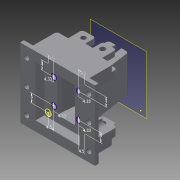
# Autodesk Inventor part: kraken_mount2
Saved by Autodesk Inventor 2014 (Build 180170000, 170)
## iProperties
Created: 2014-01-02
Part Number: kraken_mount2
Material: Generic
Document SubType Name: Modeling
Designer: stephen
Density: 1 g/cm^3
Appearance: Default
Author: stephen
Autodesk Inventor part; units mm, degrees
ref_plane "YZ Plane" through (0, 0, 0) normal (1, 0, 0) x (0, 1, 0)
ref_plane "XZ Plane" through (0, 0, 0) normal (0, 1, 0) x (-1, 0, 0)
ref_plane "XY Plane" through (0, 0, 0) normal (0, 0, 1) x (1, 0, 0)
sketch "Sketch1" plane through (0, 0, 0) normal (0, 1, 0) x (-1, 0, 0)
  line L0 (0, 0) -> (35.3, 0)
  line L1 (35.3, 0) -> (35.3, 40.3)
  line L2 (35.3, 40.3) -> (0, 40.3)
  line L3 (0, 40.3) -> (0, 0)
  line L4 (40.3, 45.3) -> (40.3, -5)
  line L5 (40.3, -5) -> (-5, -5)
  line L6 (-5, -5) -> (-5, 45.3)
  line L7 (-5, 45.3) -> (40.3, 45.3)
  dimension "d0" = 35.3
  dimension "d1" = 40.3
  dimension "d2" = 5
  constraints: 16 end point, 4 parallel, 2 perpendicular, 1 horizontal, 3 other
  measures "d0" distance of L2.end L1.end
  measures "d1" distance of L1.end L0.end
  measures "d2" distance between parallel lines of L6 L3
extrude "Extrusion1" add sketch "Sketch1" along normal blind 8
sketch "Sketch2" plane through (0, 8, 0) normal (0, 1, 0) x (1, 0, 0)
  line L0 (0, 0) -> (0, -40.3) projected
  line L1 (0, -40.3) -> (-35.3, -40.3) projected
  line L2 (-35.3, -40.3) -> (-35.3, 0) projected
  line L3 (-35.3, 0) -> (0, 0) projected
  line L4 (-32.2, -5.9) -> (-32.2, -35.2)
  line L5 (-29.8, -37.6) -> (-5.5, -37.6)
  line L6 (-3.1, -35.2) -> (-3.1, -5.9)
  circle A0 centre (-32.2, -3.5) radius 2.4
  circle A1 centre (-3.1, -3.5) radius 2.4
  circle A2 centre (-3.1, -37.6) radius 2.4
  circle A3 centre (-32.2, -37.6) radius 2.4
  line L7 (-5.5659, -5.5659) -> (-5.5659, -34.7341)
  line L8 (-5.5659, -34.7341) -> (-29.7341, -34.7341)
  line L9 (-29.7341, -34.7341) -> (-29.7341, -5.5659)
  line L10 (-29.7341, -5.5659) -> (-5.5659, -5.5659)
  line L11 (-5.5, -3.5) -> (-5.5659, -3.5)
  line L12 (-29.7341, -3.5) -> (-29.8, -3.5)
  dimension "d6" = 4.8
  dimension "d7" = 4.8
  dimension "d8" = 4.8
  dimension "d9" = 4.8
  dimension "d17" = 5.5659
  constraints: 18 end point, 8 point on circle, 4 centre point, 2 point on line, 3 other
  measures "d6" diameter of A0
  measures "d7" diameter of A1
  measures "d8" diameter of A2
  measures "d9" diameter of A3
  measures "d17" distance between parallel lines of L2 L9
extrude "Extrusion2" add sketch "Sketch2" against normal blind 4
sketch "Sketch3" plane through (0, 0, 0) normal (0, -1, 0) x (1, 0, 0)
  line L0 (-40.3, 45.3) -> (-40.3, -5) projected
  line L1 (-40.3, -5) -> (5, -5) projected
  line L2 (4.73, -7.79) -> (-40.03, -7.79)
  line L3 (-40.03, 48.09) -> (4.73, 48.09)
  line L4 (83.85, 15.65) -> (86.85, 15.65)
  circle A0 centre (25.35, 55.15) radius 2.5
  arc A1 (-22.4416, -21.2786) -> (-24.3582, -19.85) centre (-24.3582, -21.85) ccw
  line L5 (66.85, 24.65) -> (63.85, 24.65)
  line L6 (86.85, 10.65) -> (83.85, 10.65)
  circle A2 centre (25.35, 41.15) radius 2.5
  arc A3 (32.35, 38.15) -> (37.35, 33.15) centre (37.35, 38.15) ccw
  line L7 (2.35, 5.15) -> (2.35, 35.15)
  arc A4 (50.35, 7.15) -> (50.5801, 7.1553) centre (50.35, 12.15) ccw
  line L8 (-37.65, 35.15) -> (-37.65, 5.15)
  arc A5 (48.35, 26.15) -> (48.35, 30.15) centre (48.35, 28.15) ccw
  arc A6 (-22.4416, -21.2786) -> (-12.8584, -21.2786) centre (-17.65, -19.85) ccw
  line L9 (83.85, 43.65) -> (86.85, 43.65)
  line L10 (77.85, 41.65) -> (77.85, 38.15)
  arc A7 (86.85, 38.65) -> (86.85, 43.65) centre (86.85, 41.15) ccw
  line L11 (72.85, 33.15) -> (50.5801, 33.15)
  arc A8 (66.85, 24.65) -> (66.85, 29.65) centre (66.85, 27.15) ccw
  circle A9 centre (-42.65, 40.15) radius 2.1
  circle A10 centre (25.35, -14.85) radius 2.5
  arc A11 (83.85, 15.65) -> (83.85, 10.65) centre (83.85, 13.15) ccw
  line L12 (50.5801, 7.15) -> (72.85, 7.15)
  arc A12 (87.85, -6.35) -> (92.85, -1.35) centre (87.85, -1.35) ccw
  circle A13 centre (7.35, 40.15) radius 2.1
  line L13 (-47.65, 0.15) -> (-47.65, 40.15)
  arc A14 (92.85, 41.65) -> (87.85, 46.65) centre (87.85, 41.65) ccw
  arc A15 (66.85, 10.65) -> (66.85, 15.65) centre (66.85, 13.15) ccw
  line L14 (83.85, 29.65) -> (86.85, 29.65)
  line L15 (66.85, 10.65) -> (63.85, 10.65)
  arc A16 (-12.8584, 61.5786) -> (-10.9418, 60.15) centre (-10.9418, 62.15) ccw
  line L16 (83.85, 1.65) -> (86.85, 1.65)
  arc A17 (63.85, 15.65) -> (63.85, 10.65) centre (63.85, 13.15) ccw
  line L17 (48.35, 14.15) -> (38.35, 14.15)
  line L18 (-10.9418, 60.15) -> (27.35, 60.15)
  circle A18 centre (7.35, 0.15) radius 2.1
  line L19 (86.85, -3.35) -> (83.85, -3.35)
  line L20 (92.85, -1.35) -> (92.85, 41.65)
  arc A19 (86.85, -3.35) -> (86.85, 1.65) centre (86.85, -0.85) ccw
  line L21 (38.35, 10.15) -> (48.35, 10.15)
  arc A20 (82.85, 46.65) -> (77.85, 41.65) centre (82.85, 41.65) ccw
  arc A21 (86.85, 24.65) -> (86.85, 29.65) centre (86.85, 27.15) ccw
  line L22 (27.35, -19.85) -> (-10.9418, -19.85)
  arc A22 (-27.65, 60.15) -> (-47.65, 40.15) centre (-27.65, 40.15) ccw
  arc A23 (-10.9418, -19.85) -> (-12.8584, -21.2786) centre (-10.9418, -21.85) ccw
  line L23 (87.85, 46.65) -> (82.85, 46.65)
  arc A24 (48.35, 10.15) -> (48.35, 14.15) centre (48.35, 12.15) ccw
  circle A25 centre (-17.65, -19.85) radius 2.6
  line L24 (32.35, -14.85) -> (32.35, 2.15)
  arc A26 (83.85, 1.65) -> (83.85, -3.35) centre (83.85, -0.85) ccw
  arc A27 (86.85, 10.65) -> (86.85, 15.65) centre (86.85, 13.15) ccw
  circle A28 centre (25.35, 27.15) radius 2.5
  arc A29 (37.35, 7.15) -> (32.35, 2.15) centre (37.35, 2.15) ccw
  circle A30 centre (25.35, -0.85) radius 2.5
  line L25 (-27.65, 60.15) -> (-24.3582, 60.15)
  line L26 (-24.3582, -19.85) -> (-27.65, -19.85)
  line L27 (38.35, 26.15) -> (48.35, 26.15)
  circle A31 centre (-37.65, -12.85) radius 1.75
  line L28 (50.5801, 33.15) -> (50.5801, 33.1447)
  arc A32 (-17.8261, 55.1531) -> (-18.8441, 55.2947) centre (-17.65, 60.15) ccw
  arc A33 (72.85, 33.15) -> (77.85, 38.15) centre (72.85, 38.15) ccw
  arc A34 (38.35, 14.15) -> (38.35, 10.15) centre (38.35, 12.15) ccw
  arc A35 (83.85, 43.65) -> (83.85, 38.65) centre (83.85, 41.15) ccw
  line L29 (82.85, -6.35) -> (87.85, -6.35)
  circle A36 centre (2.35, 53.15) radius 1.75
  arc A37 (2.35, 35.15) -> (-37.65, 35.15) centre (-17.65, 35.15) ccw
  arc A38 (50.5801, 33.1447) -> (50.35, 33.15) centre (50.35, 28.15) ccw
  arc A39 (63.85, 29.65) -> (63.85, 24.65) centre (63.85, 27.15) ccw
  circle A40 centre (25.35, 13.15) radius 2.5
  arc A41 (77.85, -1.35) -> (82.85, -6.35) centre (82.85, -1.35) ccw
  circle A42 centre (-42.65, 20.15) radius 2.1
  arc A43 (-24.3582, 60.15) -> (-22.4416, 61.5786) centre (-24.3582, 62.15) ccw
  arc A44 (38.35, 30.15) -> (38.35, 26.15) centre (38.35, 28.15) ccw
  arc A45 (83.85, 29.65) -> (83.85, 24.65) centre (83.85, 27.15) ccw
  line L30 (50.35, 33.15) -> (37.35, 33.15)
  line L31 (50.35, 7.15) -> (37.35, 7.15)
  arc A46 (27.35, -19.85) -> (32.35, -14.85) centre (27.35, -14.85) ccw
  line L32 (86.85, 24.65) -> (83.85, 24.65)
  line L33 (50.5801, 7.1553) -> (50.5801, 7.15)
  circle A47 centre (7.35, 20.15) radius 2.1
  arc A48 (-37.65, 5.15) -> (2.35, 5.15) centre (-17.65, 5.15) ccw
  line L34 (63.85, 29.65) -> (66.85, 29.65)
  line L35 (48.35, 30.15) -> (38.35, 30.15)
  line L36 (77.85, 2.15) -> (77.85, -1.35)
  circle A49 centre (-17.65, 60.15) radius 2.6
  circle A50 centre (48.35, 20.15) radius 1.25
  line L37 (63.85, 15.65) -> (66.85, 15.65)
  arc A51 (-47.65, 0.15) -> (-27.65, -19.85) centre (-27.65, 0.15) ccw
  circle A52 centre (2.35, -12.85) radius 1.75
  arc A53 (32.35, 55.15) -> (27.35, 60.15) centre (27.35, 55.15) ccw
  arc A54 (77.85, 2.15) -> (72.85, 7.15) centre (72.85, 2.15) ccw
  circle A55 centre (-37.65, 53.15) radius 1.75
  circle A56 centre (-42.65, 0.15) radius 2.1
  line L38 (32.35, 38.15) -> (32.35, 55.15)
  line L39 (86.85, 38.65) -> (83.85, 38.65)
  circle A57 centre (38.35, 20.15) radius 1.25
  line L40 (-40.03, 48.09) -> (-47.6486, 48.09)
  line L41 (-47.6486, 48.09) -> (-47.6486, -7.79)
  line L42 (-47.6486, -7.79) -> (-40.03, -7.79)
  line L43 (4.73, 48.09) -> (12.35, 48.09)
  line L44 (12.35, 48.09) -> (12.35, -7.79)
  line L45 (12.35, -7.79) -> (4.73, -7.79)
  circle A58 centre (7.35, 40.15) radius 2.1
  circle A59 centre (7.35, 20.15) radius 2.1
  circle A60 centre (7.35, 0.15) radius 2.1
  circle A61 centre (-42.65, 40.15) radius 2.1
  circle A62 centre (-42.65, 0.15) radius 2.1
  circle A63 centre (-42.65, 20.15) radius 2.1
  line L46 (-40.3, 45.3) -> (5, 45.3)
  line L47 (5, 45.3) -> (5, -5)
  line L48 (5, -5) -> (-40.3, -5)
  line L49 (-40.3, -5) -> (-40.3, 45.3)
  line L50 (-47.6486, 48.09) -> (12.35, 48.09)
  line L51 (12.35, 48.09) -> (12.35, -7.79)
  line L52 (12.35, -7.79) -> (-47.6486, -7.79)
  line L53 (-47.6486, -7.79) -> (-47.6486, 48.09)
  point P0 (6.3945, 46.914)
  dimension "d12" = 7.62
  constraints: 104 end point, 81 tangent, 76 point on circle, 64 centre point, 55 equal radius, 26 parallel, 11 perpendicular, 6 coincident, 4 horizontal, 1 collinear, 1 concentric
  measures "d12" distance of L45.start L45.end
extrude "Extrusion3" add sketch "Sketch3" along normal blind 3 contours L0 L1 A48 L2 L42 A51 L13 A22 L40 L3 A37 L46 | A37 L3 L46 | L1 A48 L2 | A37 L3 L43 L44 L45 L2 A48 L1 L47 L46 | A22 L41 L40 | L42 L41 A51
sketch "Sketch5" plane through (0, -3, 0) normal (0, -1, 0) x (1, 0, 0)
  line L0 (-40.3, 45.3) -> (5, 45.3) projected
  line L1 (5, 45.3) -> (5, -5) projected
  line L2 (5, -5) -> (-40.3, -5) projected
  line L3 (-40.3, -5) -> (-40.3, 45.3) projected
  line L4 (0, 0) -> (-35.3, 0)
  line L5 (-35.3, 0) -> (-35.3, 40.3)
  line L6 (-35.3, 40.3) -> (0, 40.3)
  line L7 (0, 40.3) -> (0, 0)
  dimension "d15" = 35.3
  dimension "d16" = 40.3
  constraints: 8 end point, 2 parallel, 1 horizontal, 1 perpendicular
  measures "d15" distance of L5.end L6.end
  measures "d16" distance of L4.end L5.end
extrude "Extrusion4" add sketch "Sketch5" against normal up to next
sketch "Sketch6" plane through (0, 0, 0) normal (0, 1, 0) x (1, 0, 0)
  line L0 (-40.3, 5) -> (5, 5) projected
  line L1 (-47.6486, 7.79) -> (12.35, 7.79) projected
  line L2 (5, 5) -> (5, 23.7794)
  line L3 (5, 5) -> (23.7794, 5) construction
  line L4 (-40.3, 5) -> (-40.3, 33.7756)
  line L5 (-40.3, 7.79) -> (5, 7.79)
  line L6 (-40.3, 5) -> (5, 5)
  point P0 (0, 0)
  dimension "d20" = 90
  constraints: 10 end point, 4 point on line, 2 perpendicular, 1 collinear, 1 horizontal
  measures "d20" angle of L3 L2
extrude "Extrusion5" add sketch "Sketch6" along normal up to surface (8 mm away)
sketch "Sketch7" plane through (0, 0, 0) normal (0, 1, 0) x (1, 0, 0)
  line L0 (5, -45.3) -> (-40.3, -45.3) projected
  line L1 (12.35, -48.09) -> (-47.6486, -48.09) projected
  line L2 (5, 7.79) -> (12.35, 7.79) projected
  line L3 (-40.3, -45.3) -> (-40.3, -52.0309)
  line L4 (5, -45.3) -> (5, -53.1235)
  line L5 (5, -48.09) -> (-40.3, -48.09)
  line L6 (-40.3, -45.3) -> (5, -45.3)
  point P0 (0, 0)
  constraints: 8 end point, 4 point on line, 1 collinear, 1 parallel, 1 perpendicular
extrude "Extrusion6" add sketch "Sketch7" along normal up to surface (8 mm away)
sketch "Sketch8" plane through (0, 8, 0) normal (0, 1, 0) x (1, 0, 0)
  line L0 (-40.3, 7.79) -> (-40.3, -48.09) projected
  line L1 (5, -48.09) -> (5, 7.79) projected
  line L2 (5, 7.79) -> (-40.3, 7.79) projected
  line L3 (-40.3, 3.35) -> (5, 3.35)
  line L4 (5, -43.3291) -> (-40.3, -43.3291)
  point P0 (0, 0)
  dimension "d25" = 4.44
  constraints: 4 end point, 4 point on line, 2 perpendicular
  measures "d25" distance between parallel lines of L2 L3
extrude "Extrusion7" add sketch "Sketch8" along normal blind 27 contours L2 L1 L3 L0
sketch "Sketch9" plane through (0, 8, 0) normal (0, 1, 0) x (1, 0, 0)
  line L0 (-40.3, 3.35) -> (-40.3, -48.09) projected
  line L1 (-40.3, -48.09) -> (5, -48.09) projected
  line L2 (5, -48.09) -> (5, 3.35) projected
  line L3 (-40.3, -43.65) -> (5, -43.65)
  point P0 (0, 0)
  dimension "d28" = 4.44
  constraints: 2 end point, 2 point on line, 1 perpendicular
  measures "d28" distance between parallel lines of L1 L3
extrude "Extrusion8" add sketch "Sketch9" along normal blind 27
sketch "Sketch10" plane through (0, 8, 0) normal (0, 1, 0) x (1, 0, 0)
  line L0 (5, -43.65) -> (5, 3.35) projected
  line L1 (5, 3.35) -> (-40.3, 3.35) projected
  line L2 (-40.3, 3.35) -> (-40.3, -43.65) projected
  line L3 (-29.7341, -5.5659) -> (-5.5659, -5.5659) projected
  line L4 (-29.7341, -34.7341) -> (-29.7341, -5.5659) projected
  circle A0 centre (-3.1, -3.5) radius 2.4 projected
  circle A1 centre (-32.2, -3.5) radius 2.4 projected
  arc A2 (0.8686, -3) -> (-6.5252, -5.5659) centre (-3.1, -3.5) ccw
  line L5 (0.8686, -3) -> (5, -3)
  arc A3 (-27.4314, -3) -> (-36.9572, -2.9007) centre (-32.2, -3.5) ccw
  arc A4 (-29.7341, -6.9252) -> (-28.5197, -5.5659) centre (-32.2, -3.5) ccw
  line L6 (-40.3, -2.9007) -> (-36.9572, -2.9007)
  line L7 (-27.4314, -3) -> (-7.0686, -3)
  line L8 (-40.3, -2.9007) -> (-40.3, 3.35)
  line L9 (5, 3.35) -> (5, -3)
  line L10 (5, 3.35) -> (-40.3, 3.35)
  point P0 (0, 0)
  dimension "d33" = 8
  constraints: 12 end point, 7 point on circle, 5 point on line, 3 centre point, 3 collinear, 3 perpendicular, 2 coincident
  measures "d33" diameter of A2
extrude "Extrusion9" add sketch "Sketch10" along normal blind 14.274 contours L5 A2 L7 A3 L6 L2 L1 L0
sketch "Sketch11" plane through (0, 8, 0) normal (0, 1, 0) x (1, 0, 0)
  circle A0 centre (-3.1, -37.6) radius 2.4 projected
  circle A1 centre (-32.2, -37.6) radius 2.4 projected
  line L0 (-5.5659, -34.7341) -> (-29.7341, -34.7341) projected
  line L1 (-40.3, -2.9007) -> (-40.3, -43.65) projected
  line L2 (-40.3, -43.65) -> (5, -43.65) projected
  line L3 (5, -43.65) -> (5, -3) projected
  arc A2 (-36.1686, -38.1) -> (-28.2314, -38.1) centre (-32.2, -37.6) ccw
  arc A3 (-5.8905, -34.7341) -> (0.8686, -38.1) centre (-3.1, -37.6) ccw
  line L4 (0.8686, -38.1) -> (5, -38.1)
  line L5 (-40.3, -38.1) -> (-36.1686, -38.1)
  line L6 (-28.2314, -38.1) -> (-7.0686, -38.1)
  line L7 (-40.3, -38.1) -> (-40.3, -43.65)
  line L8 (-40.3, -43.65) -> (5, -43.65)
  line L9 (5, -38.1) -> (5, -43.65)
  line L10 (5, -43.65) -> (-40.3, -43.65)
  point P0 (0, 0)
  dimension "d37" = 8
  dimension "d38" = 8
  constraints: 14 end point, 5 point on circle, 4 perpendicular, 3 collinear, 3 point on line, 2 centre point, 2 coincident
  measures "d37" diameter of A2
  measures "d38" diameter of A3
extrude "Extrusion10" add sketch "Sketch11" along normal blind 14.274 contours L5 A2 L6 A3 L4 L3 L2 L1
sketch "Sketch12" plane through (12.35, 0, -7.79) normal (0, 0, -1) x (-1, 0, 0)
  line L0 (52.65, 0) -> (52.65, 35) projected
  line L1 (7.35, 35) -> (52.65, 35) projected
  line L2 (59.9986, 0) -> (59.9986, -3) projected
  line L3 (52.65, 22.6559) -> (44.6903, 22.6559)
  circle A0 centre (37.6995, 25.5722) radius 1.967
  circle A1 centre (22.3005, 25.5722) radius 1.967
  line L4 (27.8781, 10.4279) -> (122.5324, 10.4279)
  line L5 (24.2675, 25.5722) -> (35.7325, 25.5722)
  line L6 (82.6836, 13.3441) -> (74.9841, 13.3441)
  line L7 (31, 25.5722) -> (31, 22.6559)
  line L8 (74.9841, 13.3441) -> (77.9003, 13.3441) construction
  line L9 (30, 35) -> (30, 21.9681)
  line L10 (44.6903, 22.6559) -> (30, 22.6559)
  point P0 (12.35, 0)
  dimension "d41" = 90
  dimension "d67" = 7.6995
  constraints: 16 end point, 4 perpendicular, 3 point on line, 2 horizontal alignment, 1 horizontal, 1 midpoint, 1 parallel, 4 other
  measures "d41" angle of L7 L8
  measures "d67" distance from line of L9 point (37.699, 25.572)
extrude "Extrusion11" cut sketch "Sketch12" against normal through all contours A0
sketch "Sketch13" plane through (12.35, 0, -7.79) normal (0, 0, -1) x (-1, 0, 0)
  circle A0 centre (37.7, 17.5722) radius 2.2225
  circle A1 centre (22.3, 25.5722) radius 2.15
  line L0 (23.523, 25.5722) -> (36.477, 25.5722)
  line L1 (30, 25.5722) -> (30, 14.2772)
  line L2 (30, 27) -> (30, 13.5)
  line L3 (59.9986, -3) -> (0, -3) projected
  point P0 (12.35, 0)
  point P1 (30, 14.2772)
  dimension "d66" = 7.7
  dimension "d68" = 7.7
  dimension "d69" = 4.445
  dimension "d70" = 4.3
  dimension "d159" = 28.5722
  dimension "d160" = 28.5722
  constraints: 6 end point, 2 centre point, 1 midpoint, 1 point on line
  measures "d66" distance from line of L2 A0.centre
  measures "d68" distance from line of A1.centre L2
  measures "d69" diameter of A0
  measures "d70" diameter of A1
  measures "d159" distance between parallel lines of L3 L0
  measures "d160" distance from line of L3 A1.centre
extrude "Extrusion12" cut sketch "Sketch13" against normal through all contours A1
sketch "Sketch14" plane through (12.35, 0, -7.79) normal (0, 0, -1) x (-1, 0, 0)
  line L0 (52.65, 0) -> (52.65, 35) projected
  line L1 (7.35, 35) -> (52.65, 35) projected
  line L2 (7.35, 0) -> (7.35, 35) projected
  line L3 (7.35, 22.1501) -> (16.35, 22.1501)
  line L4 (16.35, 22.1501) -> (16.35, 30.6508)
  line L5 (16.35, 30.6508) -> (43.65, 30.6508)
  line L6 (43.65, 22.1501) -> (43.65, 30.6508)
  line L7 (16.35, 30.6508) -> (43.65, 30.6508)
  line L8 (43.65, 30.6508) -> (43.65, 22.1501)
  line L9 (16.35, 22.1501) -> (16.35, 30.6508)
  line L10 (7.35, 22.1501) -> (16.35, 22.1501)
  line L11 (43.65, 22.1501) -> (52.65, 22.1501)
  line L12 (59.9986, -3) -> (0, -3) projected
  point P0 (12.35, 0)
  point P1 (16.35, 35)
  point P2 (43.65, 27)
  dimension "d46" = 9
  dimension "d158" = 33.6508
  dimension "d161" = 12.8499
  dimension "d162" = 12.8499
  constraints: 18 end point, 5 perpendicular, 3 point on line, 1 horizontal, 1 parallel
  measures "d46" distance of L3.end L3.start
  measures "d158" distance between parallel lines of L12 L5
  measures "d161" distance between parallel lines of L1 L3
  measures "d162" distance between parallel lines of L1 L11
extrude "Extrusion13" cut sketch "Sketch14" against normal through all
sketch "Sketch15" plane through (12.35, 0, -7.79) normal (0, 0, -1) x (-1, 0, 0)
  line L0 (52.65, 0) -> (52.65, 22.1501) projected
  line L1 (43.65, 22.1501) -> (52.65, 22.1501)
  line L2 (52.65, 22.1501) -> (52.65, 19.1501)
  line L3 (52.65, 19.1501) -> (43.65, 19.1501)
  line L4 (43.65, 19.1501) -> (43.65, 22.1501)
  point P0 (12.35, 0)
  dimension "d52" = 3
  constraints: 8 end point, 2 parallel, 1 horizontal, 1 perpendicular, 1 point on line
  measures "d52" distance of L1.end L2.end
extrude "Extrusion14" cut sketch "Sketch15" against normal blind 4.774
sketch "Sketch16" plane through (12.35, 0, -7.79) normal (0, 0, -1) x (-1, 0, 0)
  line L0 (7.35, 22.1501) -> (16.35, 22.1501)
  line L1 (16.35, 22.1501) -> (16.35, 19.1501)
  line L2 (16.35, 19.1501) -> (7.35, 19.1501)
  line L3 (7.35, 19.1501) -> (7.35, 22.1501)
  point P0 (12.35, 0)
  dimension "d55" = 3
  constraints: 8 end point, 2 parallel, 1 horizontal, 1 perpendicular
  measures "d55" distance of L0.end L1.end
extrude "Extrusion15" cut sketch "Sketch16" against normal blind 4.774
sketch "Sketch17" plane through (5, 0, 48.09) normal (0, 0, 1) x (1, 0, 0)
  line L0 (-45.3, 22.1501) -> (-36.3, 22.1501)
  line L1 (-36.3, 22.1501) -> (-36.3, 19.1501)
  line L2 (-36.3, 19.1501) -> (-45.3, 19.1501)
  line L3 (-45.3, 19.1501) -> (-45.3, 22.1501)
  point P0 (-5, 0)
  dimension "d58" = 3
  constraints: 8 end point, 2 parallel, 1 horizontal, 1 perpendicular
  measures "d58" distance of L0.end L1.end
extrude "Extrusion16" cut sketch "Sketch17" against normal blind 4.774
sketch "Sketch18" plane through (5, 0, 48.09) normal (0, 0, 1) x (1, 0, 0)
  line L0 (0, 0) -> (0, 22.1501) projected
  line L1 (-9, 22.1501) -> (0, 22.1501)
  line L2 (0, 22.1501) -> (0, 19.1501)
  line L3 (0, 19.1501) -> (-9, 19.1501)
  line L4 (-9, 19.1501) -> (-9, 22.1501)
  point P0 (-5, 0)
  dimension "d61" = 3
  constraints: 8 end point, 2 parallel, 1 horizontal, 1 perpendicular, 1 point on line
  measures "d61" distance of L1.end L2.end
extrude "Extrusion17" cut sketch "Sketch18" against normal blind 4.774
fillet "Fillet4" radius 2 8 edges at (-31.3, 30.6508, -5.57) (-40.3, 19.1501, -5.403) (-40.3, 8, 20.5003) (-40.3, 22.1501, -0.0577) (-4, 30.6508, -5.57) (5, 19.1501, -5.403) (5, 22.1501, -0.008) (5, 8, 20.55)
fillet "Fillet5" radius 2 6 edges at (-40.3, 19.1501, 45.703) (-40.3, 22.1501, 40.708) (-31.3, 30.6508, 45.87) (5, 19.1501, 45.703) (5, 22.1501, 40.708) (-4, 30.6508, 45.87)
sketch "Sketch19" plane through (0, 8, 0) normal (0, 1, 0) x (1, 0, 0)
  line L0 (-29.7341, -34.7341) -> (-29.7341, -5.5659) projected
  line L1 (-29.7341, -34.7341) -> (-29.7341, -5.5659)
  line L2 (-29.7341, -5.5659) -> (-24.7341, -5.5659)
  line L3 (-24.7341, -5.5659) -> (-24.7341, -34.7341)
  line L4 (-24.7341, -34.7341) -> (-29.7341, -34.7341)
  point P0 (0, 0)
  dimension "d71" = 5
  constraints: 8 end point, 3 equal length, 1 perpendicular
  measures "d71" distance of L0.end L2.end
extrude "Extrusion18" add sketch "Sketch19" against normal blind 4
sketch "Sketch20" plane through (0, 8, 0) normal (0, 1, 0) x (1, 0, 0)
  line L0 (-5.5659, -5.5659) -> (-5.5659, -34.7341) projected
  line L1 (-5.5659, -34.7341) -> (-5.5659, -5.5659)
  line L2 (-5.5659, -5.5659) -> (-10.5659, -5.5659)
  line L3 (-10.5659, -5.5659) -> (-10.5659, -34.7341)
  line L4 (-10.5659, -34.7341) -> (-5.5659, -34.7341)
  point P0 (0, 0)
  dimension "d74" = 5
  constraints: 8 end point, 3 equal length, 1 perpendicular
  measures "d74" distance of L2.end L0.start
extrude "Extrusion19" add sketch "Sketch20" against normal blind 4
sketch "Sketch21" plane through (0, 4, 0) normal (0, -1, 0) x (1, 0, 0)
  circle A0 centre (-32.2, 37.6) radius 2.4 projected
  circle A1 centre (-3.1, 37.6) radius 2.4 projected
  circle A2 centre (-3.1, 3.5) radius 2.4 projected
  circle A3 centre (-32.2, 3.5) radius 2.4 projected
  circle A4 centre (-27.7, 30.6) radius 2.165
  circle A5 centre (-27.7, 10.5) radius 2.165
  circle A6 centre (-7.6, 10.5) radius 2.165
  circle A7 centre (-7.6, 30.6) radius 2.165
  dimension "d77" = 4.33
  dimension "d78" = 4.5
  dimension "d79" = 7
  dimension "d94" = 4.33
  dimension "d95" = 4.33
  dimension "d96" = 4.33
  dimension "d97" = 4.5
  dimension "d98" = 7
  dimension "d99" = 7
  dimension "d100" = 4.5
  dimension "d101" = 7
  dimension "d102" = 4.5
  constraints: 4 centre point
  measures "d77" diameter of A4
  measures "d78" horizontal distance of A0.centre A4.centre
  measures "d79" vertical distance of A0.centre A4.centre
  measures "d94" diameter of A5
  measures "d95" diameter of A6
  measures "d96" diameter of A7
  measures "d97" horizontal distance of A5.centre A3.centre
  measures "d98" vertical distance of A5.centre A3.centre
  measures "d99" vertical distance of A2.centre A6.centre
  measures "d100" horizontal distance of A6.centre A2.centre
  measures "d101" vertical distance of A1.centre A7.centre
  measures "d102" horizontal distance of A7.centre A1.centre
ref_plane "Work Plane1" through (0, 46, 0) normal (0, 1, 0) x (1, 0, 0)
sketch "Sketch55" plane through (0, 8, 0) normal (0, 1, 0) x (1, 0, 0)
  line L0 (-24.7341, -5.5659) -> (-10.5659, -5.5659) projected
  line L1 (-10.5659, -5.5659) -> (-10.5659, -34.7341) projected
  line L2 (-10.5659, -5.5659) -> (-10.5659, -34.7341)
  line L3 (-10.5659, -34.7341) -> (-4.9659, -34.7341)
  line L4 (-4.9659, -34.7341) -> (-4.9659, -5.5659)
  line L5 (-4.9659, -5.5659) -> (-10.5659, -5.5659)
  point P0 (0, 0)
  dimension "d163" = 5.6
  constraints: 8 end point, 2 parallel, 2 perpendicular
  measures "d163" distance of L3.end L1.end
sketch "Sketch57" plane through (0, 46, 0) normal (0, 1, 0) x (1, 0, 0)
  line L0 (-22.3184, -11.5622) -> (-12.9154, -11.5622)
  line L1 (-12.9154, -11.5622) -> (-12.9154, -27.5403)
  line L2 (-12.9154, -27.5403) -> (-22.3184, -27.5403)
  line L3 (-22.3184, -27.5403) -> (-22.3184, -11.5622)
  point P0 (0, 0)
  constraints: 8 end point, 2 parallel, 1 horizontal, 1 perpendicular
sketch3d "3D Sketch19"
  line L0 (-7.6, 4, 10.5) -> (-12.9154, 46, 11.5622)
sweep "Sweep14" add profiles "Sketch55" path "3D Sketch19"
sketch "Sketch58" plane through (0, 8, 0) normal (0, 1, 0) x (1, 0, 0)
  line L0 (-10.5659, -34.7341) -> (-24.7341, -34.7341) projected
  line L1 (-24.7341, -5.5659) -> (-30.3341, -5.5659)
  line L2 (-30.3341, -5.5659) -> (-30.3341, -34.7341)
  line L3 (-30.3341, -34.7341) -> (-24.7341, -34.7341)
  line L4 (-24.7341, -34.7341) -> (-24.7341, -5.5659)
  point P0 (0, 0)
  dimension "d165" = 5.6
  constraints: 8 end point, 2 parallel, 1 horizontal, 1 perpendicular, 1 point on line
  measures "d165" distance of L3.end L2.end
sketch3d "3D Sketch20"
  line L0 (-27.7, 4, 10.5) -> (-22.3184, 46, 11.5622)
sweep "Sweep15" add profiles "Sketch58" path "3D Sketch20"
sketch3d "3D Sketch21"
  line L0 (-27.7, 4, 30.6) -> (-22.3184, 46, 27.5403)
sweep "Sweep16" cut profiles "Sketch21" path "3D Sketch21" contours A4
sketch3d "3D Sketch22"
  line L0 (-27.7, 4, 10.5) -> (-22.3184, 46, 11.5622)
sweep "Sweep17" cut profiles "Sketch21" path "3D Sketch22" contours A5
sketch3d "3D Sketch23"
  line L0 (-7.6, 4, 30.6) -> (-12.9154, 46, 27.5403)
sweep "Sweep18" cut profiles "Sketch21" path "3D Sketch23" contours A7
sketch3d "3D Sketch24"
  line L0 (-7.6, 4, 10.5) -> (-12.9154, 46, 11.5622)
sweep "Sweep19" cut profiles "Sketch21" path "3D Sketch24" contours A6
fillet "Fillet10" radius 2 2 edges at (-24.7341, 8, 20.15) (-9.775, 46, 21.111)
fillet "Fillet11" radius 2 1 edges at (-25.465, 46, 21.111)
sketch "Sketch65" plane through (-4, 22.274, 43.65) normal (0, 0, -1) x (-1, 0, 0)
  line L0 (0, 0) -> (27.3, 0) projected
  line L1 (25.3, 8.3768) -> (2, 8.3768) projected
  line L2 (13.65, 0) -> (16.65, 0)
  line L3 (16.65, 0) -> (16.65, 8.3768)
  line L4 (16.65, 8.3768) -> (13.65, 8.3768)
  line L5 (13.65, 0) -> (10.65, 0)
  line L6 (10.65, 0) -> (10.65, 8.3768)
  line L7 (10.65, 8.3768) -> (13.65, 8.3768)
  point P0 (-4, -22.274)
  constraints: 12 end point, 2 midpoint, 2 parallel
extrude "Extrusion31" cut sketch "Sketch65" against normal blind 10
fillet "Fillet12" radius 2 2 edges at (-14.65, 30.6508, 45.87) (-20.65, 30.6508, 45.87)
sketch "Sketch66" plane through (-31.3, 22.274, -3.35) normal (0, 0, 1) x (1, 0, 0)
  line L0 (25.3, 8.3768) -> (2, 8.3768) projected
  line L1 (0, 0) -> (27.3, 0) projected
  line L2 (13.65, 0) -> (16.65, 0)
  line L3 (16.65, 0) -> (16.65, 8.3768)
  line L4 (16.65, 8.3768) -> (13.65, 8.3768)
  line L5 (13.65, 0) -> (10.65, 0)
  line L6 (10.65, 0) -> (10.65, 8.3768)
  line L7 (10.65, 8.3768) -> (13.65, 8.3768)
  point P0 (31.3, -22.274)
  constraints: 12 end point, 2 midpoint, 2 parallel
extrude "Extrusion32" cut sketch "Sketch66" against normal blind 10
fillet "Fillet13" radius 2 2 edges at (-14.65, 30.6508, -5.57) (-20.65, 30.6508, -5.57)
body "Solid1"
